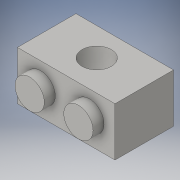
# Autodesk Inventor part: Yee_1x2BrickWithHole
Saved by Autodesk Inventor 2016 (Build 200138000, 138)
## iProperties
Created: 2018-02-11
Part Number: Yee_1x2BrickWithHole
Material: Generic
Document SubType Name: Modeling
Designer: Nathan
Density: 1 g/cm^3
Appearance: Default
Author: Nathan
Autodesk Inventor part; units mm, degrees
ref_plane "YZ Plane" through (0, 0, 0) normal (1, 0, 0) x (0, 1, 0)
ref_plane "XZ Plane" through (0, 0, 0) normal (0, 1, 0) x (-1, 0, 0)
ref_plane "XY Plane" through (0, 0, 0) normal (0, 0, 1) x (1, 0, 0)
sketch "Sketch1" plane through (0, 0, 0) normal (0, 0, 1) x (1, 0, 0)
  line L0 (0, 0) -> (16, 0)
  line L1 (16, 0) -> (16, 8)
  line L2 (16, 8) -> (0, 8)
  line L3 (0, 8) -> (0, 0)
  dimension "d0" = 16
  dimension "d1" = 8
  constraints: 8 end point, 2 parallel, 1 horizontal, 1 perpendicular
  measures "d0" distance of L2.end L1.end
  measures "d1" distance of L1.end L0.end
extrude "Extrusion1" add sketch "Sketch1" against normal blind 9.6
sketch "Sketch2" plane through (0, 0, 0) normal (0, 0, 1) x (1, 0, 0)
  circle A0 centre (3.8, 4.2) radius 2.4
  circle A1 centre (11.8, 4.2) radius 2.4
  line L0 (16, 8) -> (0, 8) projected
  line L1 (0, 0) -> (0, 8) projected
  dimension "d4" = 4.8
  dimension "d5" = 4.8
  dimension "d6" = 3.8
  dimension "d7" = 3.8
  dimension "d8" = 8
  constraints: 2 centre point, 1 horizontal alignment
  measures "d4" diameter of A0
  measures "d5" diameter of A1
  measures "d6" distance from line of L0 A0.centre
  measures "d7" distance from line of L1 A0.centre
  measures "d8" distance of A1.centre A0.centre
extrude "Extrusion2" add sketch "Sketch2" along normal blind 1.8
sketch "Sketch3" plane through (0, 0, -9.6) normal (0, 0, -1) x (-1, 0, 0)
  line L0 (-14.8, 6.8) -> (-1.2, 6.8)
  line L1 (-1.2, 6.8) -> (-1.2, 1.2)
  line L2 (-1.2, 1.2) -> (-14.8, 1.2)
  line L3 (-14.8, 1.2) -> (-14.8, 6.8)
  line L4 (-16, 8) -> (0, 8) projected
  line L5 (-16, 0) -> (-16, 8) projected
  line L6 (-16, 0) -> (0, 0) projected
  line L7 (0, 0) -> (0, 8) projected
  circle A0 centre (-8, 4) radius 1
  dimension "d11" = 1.2
  dimension "d12" = 1.2
  dimension "d13" = 1.2
  dimension "d14" = 1.2
  dimension "d15" = 2
  dimension "d16" = 8
  dimension "d17" = 4
  constraints: 8 end point, 2 parallel, 1 centre point, 1 horizontal, 1 perpendicular
  measures "d11" distance between parallel lines of L4 L0
  measures "d12" distance between parallel lines of L5 L3
  measures "d13" distance between parallel lines of L6 L2
  measures "d14" distance between parallel lines of L7 L1
  measures "d15" diameter of A0
  measures "d16" distance from line of L5 A0.centre
  measures "d17" distance from line of L6 A0.centre
extrude "Extrusion3" cut sketch "Sketch3" against normal blind 1.8 contours L0 L1 L2 L3
sketch "Sketch4" plane through (0, 8, 0) normal (0, 1, 0) x (1, 0, 0)
  line L0 (0, 9.6) -> (16, 9.6) projected
  line L1 (14.8, 7.8) -> (1.2, 7.8) projected
  line L2 (0, 0) -> (0, 9.6) projected
  point P0 (8, 5)
  dimension "d21" = 2.8
  dimension "d22" = 8
  measures "d21" distance from line of L1 point (8, 5)
  measures "d22" distance from line of L2 point (8, 5)
hole "Hole1" at (8, 8, -5) direction (0, -1, 0) diameter 4.8 depth 25.4 tip angle 118
body "Solid1"
